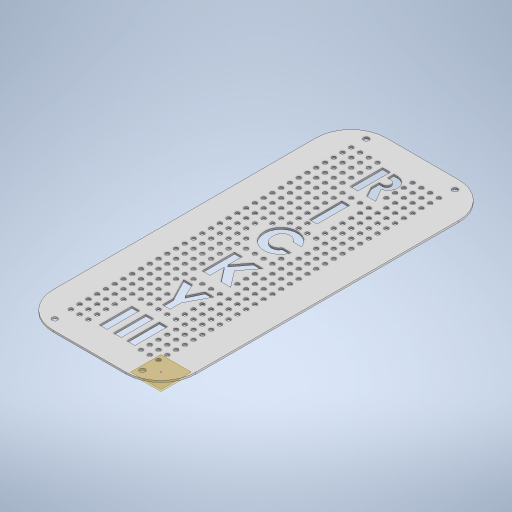
# Autodesk Inventor part: Ground Station cover
Saved by Autodesk Inventor 2023 (Build 270158000, 158)
## iProperties
Created: 2023-02-28
Part Number: Ground Station cover
Material: Generic
Document SubType Name: Modeling
Designer: mikep
Density: 1 g/cm^3
Appearance: Default
Author: mikep
Autodesk Inventor part; units mm, degrees
ref_plane "YZ Plane" through (0, 0, 0) normal (1, 0, 0) x (0, 1, 0)
ref_plane "XZ Plane" through (0, 0, 0) normal (0, 1, 0) x (-1, 0, 0)
ref_plane "XY Plane" through (0, 0, 0) normal (0, 0, 1) x (1, 0, 0)
ref_plane "Work Plane1" through (0, 12.7, 0) normal (0, 1, 0) x (1, 0, 0)
sketch "Sketch5" plane through (0, 12.7, 0) normal (0, 1, 0) x (1, 0, 0)
  line L0 (-90.805, -12.7) -> (12.7, -12.7)
  line L1 (12.7, -12.7) -> (12.7, 228.6)
  line L2 (12.7, 228.6) -> (-90.805, 228.6)
  line L3 (-90.805, 228.6) -> (-90.805, -12.7)
  line L4 (0, 0) -> (0, 215.9) projected
  line L5 (0, 215.9) -> (-78.105, 215.9) projected
  dimension "d18" = 241.3
  dimension "d19" = 103.505
  dimension "d20" = 12.7
  dimension "d21" = 12.7
  constraints: 8 end point, 2 parallel, 1 horizontal, 1 perpendicular
  measures "d18" distance of L1.end L0.end
  measures "d19" distance of L1.end L2.end
  measures "d20" distance between parallel lines of L1 L4
  measures "d21" distance between parallel lines of L5 L2
extrude "Extrusion4" add sketch "Sketch5" along normal blind 1.27
sketch "Sketch6" plane through (0, 13.97, 0) normal (0, 1, 0) x (1, 0, 0)
  point P0 (0, 0)
ref_plane "Work Plane3" through (0, 13.97, 0) normal (0, 1, 0) x (1, 0, 0)
sketch "Sketch8" plane through (0, 13.97, 0) normal (0, 1, 0) x (1, 0, 0)
  line L0 (-74.295, 3.81) -> (-3.81, 3.81) projected
  line L1 (-51.8748, 30.8065) -> (-46.268, 30.8065)
  line L2 (-46.268, 30.8065) -> (-46.268, 7.3025)
  line L3 (-46.268, 7.3025) -> (-51.8748, 7.3025)
  line L4 (-51.8748, 7.3025) -> (-51.8748, 30.8065)
  line L5 (-41.6807, 30.8065) -> (-36.074, 30.8065)
  line L6 (-36.074, 30.8065) -> (-36.074, 7.3025)
  line L7 (-36.074, 7.3025) -> (-41.6807, 7.3025)
  line L8 (-41.6807, 7.3025) -> (-41.6807, 30.8065)
  line L9 (-31.9235, 30.8065) -> (-26.0983, 30.8065)
  line L10 (-26.0983, 30.8065) -> (-26.0983, 7.3025)
  line L11 (-26.0983, 7.3025) -> (-31.9235, 7.3025)
  line L12 (-31.9235, 7.3025) -> (-31.9235, 30.8065)
  line L13 (-41.6192, 42.7474) -> (-36.1235, 42.7474)
  line L14 (-36.1235, 42.7474) -> (-36.1235, 50.6586)
  line L15 (-36.1235, 50.6586) -> (-27.9507, 66.2951)
  line L16 (-27.9507, 66.2951) -> (-34.288, 66.2951)
  line L17 (-34.288, 66.2951) -> (-38.8713, 56.5194)
  line L18 (-38.8713, 56.5194) -> (-43.4546, 66.2951)
  line L19 (-43.4546, 66.2951) -> (-49.7919, 66.2951)
  line L20 (-49.7919, 66.2951) -> (-41.6192, 50.6586)
  line L21 (-41.6192, 50.6586) -> (-41.6192, 42.7474)
  line L22 (-48.5981, 101.9465) -> (-48.5981, 78.5001)
  line L23 (-48.5981, 78.5001) -> (-42.9914, 78.5001)
  line L24 (-42.9914, 78.5001) -> (-42.9914, 88.9127)
  line L25 (-42.9914, 88.9127) -> (-34.9817, 78.5001)
  line L26 (-34.9817, 78.5001) -> (-27.9507, 78.5001)
  line L27 (-27.9507, 78.5001) -> (-36.9685, 90.2233)
  line L28 (-36.9685, 90.2233) -> (-27.9507, 101.9465)
  line L29 (-27.9507, 101.9465) -> (-34.9817, 101.9465)
  line L30 (-34.9817, 101.9465) -> (-42.9914, 91.534)
  line L31 (-42.9914, 91.534) -> (-42.9914, 101.9465)
  line L32 (-42.9914, 101.9465) -> (-48.5981, 101.9465)
  line L33 (-27.6673, 121.9946) -> (-33.9997, 121.9946)
  arc A0 (-44.2292, 129.1064) -> (-44.1364, 122.3681) centre (-36.4286, 125.844) ccw
  line L34 (-33.8768, 129.6183) -> (-27.6561, 129.6183)
  arc A1 (-44.1364, 122.3681) -> (-33.9997, 121.9946) centre (-38.9754, 124.6955) ccw
  arc A2 (-33.8768, 129.6183) -> (-44.2292, 129.1064) centre (-38.9307, 126.8905) ccw
  arc A3 (-27.6561, 129.6183) -> (-50.2579, 129.6183) centre (-38.957, 125.9562) ccw
  arc A4 (-50.2579, 129.6183) -> (-50.2881, 122.3885) centre (-38.957, 125.9562) ccw
  arc A5 (-50.2881, 122.3885) -> (-27.6673, 121.9946) centre (-38.9225, 125.3595) ccw
  line L35 (-41.8513, 173.0184) -> (-36.3002, 173.0184)
  line L36 (-36.3002, 173.0184) -> (-36.3002, 149.5617)
  line L37 (-36.3002, 149.5617) -> (-41.8513, 149.5617)
  line L38 (-41.8513, 149.5617) -> (-41.8513, 173.0184)
  line L39 (-47.9527, 208.5865) -> (-47.9527, 185.035)
  line L40 (-47.9527, 185.035) -> (-42.2829, 185.035)
  line L41 (-42.2829, 185.035) -> (-42.2829, 194.0541)
  line L42 (-39.7429, 192.064) -> (-35.8412, 185.035)
  line L43 (-35.8412, 185.035) -> (-29.3552, 185.035)
  line L44 (-29.3552, 185.035) -> (-34.8878, 194.4069)
  arc A6 (-34.8878, 194.4069) -> (-34.8878, 208.176) centre (-36.7536, 201.2914) ccw
  arc A7 (-34.8878, 208.176) -> (-37.3133, 208.5865) centre (-38.2098, 195.9186) ccw
  line L45 (-42.2829, 203.9834) -> (-42.2829, 197.929)
  line L46 (-39.7429, 197.929) -> (-37.2678, 197.929)
  line L47 (-39.7429, 203.9834) -> (-37.2678, 203.9834)
  arc A8 (-37.2678, 197.929) -> (-37.2678, 203.9834) centre (-37.2678, 200.9562) ccw
  line L48 (-42.2829, 194.0541) -> (-42.2829, 197.929)
  line L49 (-39.7429, 192.064) -> (-39.7429, 197.929)
  line L50 (-42.2829, 203.9834) -> (-42.2829, 208.5865)
  line L51 (-39.7429, 208.5865) -> (-39.7429, 203.9834)
  line L52 (-47.9527, 208.5865) -> (-42.2829, 208.5865)
  line L53 (-39.7429, 208.5865) -> (-37.3133, 208.5865)
  line L54 (-90.805, 228.6) -> (-90.805, -12.7) projected
  line L55 (-90.805, 107.95) -> (12.7, 107.95) construction
  line L56 (12.7, -12.7) -> (12.7, 228.6) projected
  line L57 (12.7, 228.6) -> (-90.805, 228.6) projected
  line L58 (-39.0525, 228.6) -> (-39.0525, -12.7) construction
  line L59 (-90.805, -12.7) -> (12.7, -12.7) projected
  point P0 (0, 0)
  point P1 (-31.9235, 3.81)
  point P2 (-51.8748, 3.81)
  point P3 (-41.6807, 3.81)
  point P4 (-26.0983, 3.81)
  point P5 (-46.268, 3.81)
  point P6 (-36.074, 3.81)
  dimension "d54" = 2.54
  dimension "d55" = 2.54
  constraints: 110 end point, 19 point on circle, 14 perpendicular, 13 parallel, 11 horizontal, 11 point on line, 9 centre point, 5 tangent, 4 equal length, 4 midpoint, 4 vertical, 1 concentric
  measures "d54" distance from line of L49 L45.end
  measures "d55" distance between parallel lines of L50 L51
extrude "Extrusion5" cut sketch "Sketch8" against normal blind 25.4 contours L1 L2 L3 L4 | L5 L6 L7 L8 | L9 L10 L11 L12 | L21 L20 L19 L18 L17 L16 L15 L14 L13 | L32 L31 L30 L29 L28 L27 L26 L25 L24 L23 L22 | A5 A4 A3 L34 A2 A0 A1 L33 | L35 L36 L37 L38 | L52 L50 L45 L48 L41 L40 L39 | L49 L46 A8 L47 L51 L53 A7 A6 L44 L43 L42
ref_plane "Work Plane2" through (0, 13.97, 0) normal (0, 1, 0) x (1, 0, 0)
sketch "Sketch9" plane through (0, 13.97, 0) normal (0, 1, 0) x (1, 0, 0)
  line L0 (-3.81, 212.09) -> (-74.295, 212.09) construction
  line L1 (-74.295, 212.09) -> (-3.81, 212.09) construction
  line L2 (-3.81, 212.09) -> (-74.295, 212.09) construction
  line L3 (-74.295, 212.09) -> (-74.295, 22.9425) construction
  line L4 (-74.295, 3.81) -> (-3.81, 3.81) construction
  line L5 (-71.9663, 3.81) -> (-6.4229, 3.81) construction
  point P0 (0, 0)
  point P1 (-71.9663, 209.9147)
  point P2 (-71.9663, 203.5647)
  point P3 (-71.9663, 197.2147)
  point P4 (-71.9663, 190.8647)
  point P5 (-71.9663, 184.5147)
  point P6 (-71.9663, 178.1647)
  point P7 (-71.9663, 171.8147)
  point P8 (-71.9663, 165.4647)
  point P9 (-71.9663, 159.1147)
  point P10 (-71.9663, 152.7647)
  point P11 (-71.9663, 146.4147)
  point P12 (-71.9663, 140.0647)
  point P13 (-71.9663, 133.7147)
  point P14 (-71.9663, 127.3647)
  point P15 (-71.9663, 121.0147)
  point P16 (-71.9663, 114.6647)
  point P17 (-71.9663, 108.3147)
  point P18 (-71.9663, 101.9647)
  point P19 (-71.9663, 95.6147)
  point P20 (-71.9663, 89.2647)
  point P21 (-71.9663, 82.9147)
  point P22 (-71.9663, 76.5647)
  point P23 (-71.9663, 70.2147)
  point P24 (-71.9663, 63.8647)
  point P25 (-71.9663, 57.5147)
  point P26 (-71.9663, 51.1647)
  point P27 (-71.9663, 44.8147)
  point P28 (-71.9663, 38.4647)
  point P29 (-71.9663, 32.1147)
  point P30 (-71.9663, 25.7647)
  point P31 (-71.9663, 19.4147)
  point P32 (-71.9663, 13.0647)
  point P33 (-71.9663, 6.7147)
  point P34 (-65.6163, 209.9147)
  point P35 (-65.6163, 203.5647)
  point P36 (-65.6163, 197.2147)
  point P37 (-65.6163, 190.8647)
  point P38 (-65.6163, 184.5147)
  point P39 (-65.6163, 178.1647)
  point P40 (-65.6163, 171.8147)
  point P41 (-65.6163, 165.4647)
  point P42 (-65.6163, 159.1147)
  point P43 (-65.6163, 152.7647)
  point P44 (-65.6163, 146.4147)
  point P45 (-65.6163, 140.0647)
  point P46 (-65.6163, 133.7147)
  point P47 (-65.6163, 127.3647)
  point P48 (-65.6163, 121.0147)
  point P49 (-65.6163, 114.6647)
  point P50 (-65.6163, 108.3147)
  point P51 (-65.6163, 101.9647)
  point P52 (-65.6163, 95.6147)
  point P53 (-65.6163, 89.2647)
  point P54 (-65.6163, 82.9147)
  point P55 (-65.6163, 76.5647)
  point P56 (-65.6163, 70.2147)
  point P57 (-65.6163, 63.8647)
  point P58 (-65.6163, 57.5147)
  point P59 (-65.6163, 51.1647)
  point P60 (-65.6163, 44.8147)
  point P61 (-65.6163, 38.4647)
  point P62 (-65.6163, 32.1147)
  point P63 (-65.6163, 25.7647)
  point P64 (-65.6163, 19.4147)
  point P65 (-65.6163, 13.0647)
  point P66 (-65.6163, 6.7147)
  point P67 (-59.2663, 209.9147)
  point P68 (-59.2663, 203.5647)
  point P69 (-59.2663, 197.2147)
  point P70 (-59.2663, 190.8647)
  point P71 (-59.2663, 184.5147)
  point P72 (-59.2663, 178.1647)
  point P73 (-59.2663, 171.8147)
  point P74 (-59.2663, 165.4647)
  point P75 (-59.2663, 159.1147)
  point P76 (-59.2663, 152.7647)
  point P77 (-59.2663, 146.4147)
  point P78 (-59.2663, 140.0647)
  point P79 (-59.2663, 133.7147)
  point P80 (-59.2663, 127.3647)
  point P81 (-59.2663, 121.0147)
  point P82 (-59.2663, 114.6647)
  point P83 (-59.2663, 108.3147)
  point P84 (-59.2663, 101.9647)
  point P85 (-59.2663, 95.6147)
  point P86 (-59.2663, 89.2647)
  point P87 (-59.2663, 82.9147)
  point P88 (-59.2663, 76.5647)
  point P89 (-59.2663, 70.2147)
  point P90 (-59.2663, 63.8647)
  point P91 (-59.2663, 57.5147)
  point P92 (-59.2663, 51.1647)
  point P93 (-59.2663, 44.8147)
  point P94 (-59.2663, 38.4647)
  point P95 (-59.2663, 32.1147)
  point P96 (-59.2663, 25.7647)
  point P97 (-59.2663, 19.4147)
  point P98 (-59.2663, 13.0647)
  point P99 (-59.2663, 6.7147)
  point P100 (-52.9163, 209.9147)
  point P101 (-52.9163, 203.5647)
  point P102 (-52.9163, 197.2147)
  point P103 (-52.9163, 190.8647)
  point P104 (-52.9163, 184.5147)
  point P105 (-52.9163, 178.1647)
  point P106 (-52.9163, 171.8147)
  point P107 (-52.9163, 165.4647)
  point P108 (-52.9163, 159.1147)
  point P109 (-52.9163, 152.7647)
  point P110 (-52.9163, 146.4147)
  point P111 (-52.9163, 140.0647)
  point P112 (-52.9163, 133.7147)
  point P113 (-52.9163, 114.6647)
  point P114 (-52.9163, 108.3147)
  point P115 (-52.9163, 101.9647)
  point P116 (-52.9163, 95.6147)
  point P117 (-52.9163, 89.2647)
  point P118 (-52.9163, 82.9147)
  point P119 (-52.9163, 76.5647)
  point P120 (-52.9163, 70.2147)
  point P121 (-52.9163, 63.8647)
  point P122 (-52.9163, 57.5147)
  point P123 (-52.9163, 51.1647)
  point P124 (-52.9163, 44.8147)
  point P125 (-52.9163, 38.4647)
  point P126 (-52.9163, 25.7647)
  point P127 (-52.9163, 19.4147)
  point P128 (-52.9163, 13.0647)
  point P129 (-52.9163, 6.7147)
  point P130 (-46.5663, 203.5647)
  point P131 (-46.5663, 197.2147)
  point P132 (-46.5663, 190.8647)
  point P133 (-46.5663, 184.5147)
  point P134 (-46.5663, 178.1647)
  point P135 (-46.5663, 171.8147)
  point P136 (-46.5663, 165.4647)
  point P137 (-46.5663, 159.1147)
  point P138 (-46.5663, 152.7647)
  point P139 (-46.5663, 146.4147)
  point P140 (-46.5663, 140.0647)
  point P141 (-46.5663, 133.7147)
  point P142 (-46.5663, 127.3647)
  point P143 (-46.5663, 121.0147)
  point P144 (-46.5663, 114.6647)
  point P145 (-46.5663, 108.3147)
  point P146 (-46.5663, 101.9647)
  point P147 (-46.5663, 95.6147)
  point P148 (-46.5663, 89.2647)
  point P149 (-46.5663, 82.9147)
  point P150 (-46.5663, 70.2147)
  point P151 (-46.5663, 63.8647)
  point P152 (-46.5663, 51.1647)
  point P153 (-46.5663, 44.8147)
  point P154 (-46.5663, 38.4647)
  point P155 (-46.5663, 25.7647)
  point P156 (-46.5663, 19.4147)
  point P157 (-46.5663, 13.0647)
  point P158 (-46.5663, 6.7147)
  point P159 (-40.2163, 203.5647)
  point P160 (-40.2163, 197.2147)
  point P161 (-40.2163, 190.8647)
  point P162 (-40.2163, 178.1647)
  point P163 (-40.2163, 171.8147)
  point P164 (-40.2163, 165.4647)
  point P165 (-40.2163, 159.1147)
  point P166 (-40.2163, 152.7647)
  point P167 (-40.2163, 146.4147)
  point P168 (-40.2163, 140.0647)
  point P169 (-40.2163, 133.7147)
  point P170 (-40.2163, 114.6647)
  point P171 (-40.2163, 108.3147)
  point P172 (-40.2163, 101.9647)
  point P173 (-40.2163, 95.6147)
  point P174 (-40.2163, 89.2647)
  point P175 (-40.2163, 82.9147)
  point P176 (-40.2163, 70.2147)
  point P177 (-40.2163, 63.8647)
  point P178 (-40.2163, 57.5147)
  point P179 (-40.2163, 51.1647)
  point P180 (-40.2163, 44.8147)
  point P181 (-40.2163, 38.4647)
  point P182 (-40.2163, 25.7647)
  point P183 (-40.2163, 19.4147)
  point P184 (-40.2163, 13.0647)
  point P185 (-40.2163, 6.7147)
  point P186 (-33.8663, 203.5647)
  point P187 (-33.8663, 197.2147)
  point P188 (-33.8663, 190.8647)
  point P189 (-33.8663, 184.5147)
  point P190 (-33.8663, 178.1647)
  point P191 (-33.8663, 140.0647)
  point P192 (-33.8663, 133.7147)
  point P193 (-33.8663, 121.0147)
  point P194 (-33.8663, 114.6647)
  point P195 (-33.8663, 108.3147)
  point P196 (-33.8663, 101.9647)
  point P197 (-33.8663, 95.6147)
  point P198 (-33.8663, 89.2647)
  point P199 (-33.8663, 82.9147)
  dimension "d48" = 6.35
  dimension "d51" = 6.35
  constraints: 8 end point, 2 horizontal, 2 point on line, 1 collinear, 1 vertical, 313 other
  measures "d48" distance of point (-71.966, 209.915) point (-71.966, 203.565)
  measures "d51" distance of point (-71.966, 209.915) point (-65.616, 209.915)
hole "Hole1" at (-65.6163, 13.97, -209.9147) at (-71.9663, 13.97, -209.9147) at (-59.2663, 13.97, -209.9147) at (-52.9163, 13.97, -209.9147) at (-27.5163, 13.97, -209.9147) at (-21.1663, 13.97, -209.9147) at (-14.8163, 13.97, -209.9147) at (-8.4663, 13.97, -209.9147) at (-8.4663, 13.97, -203.5647) at (-14.8163, 13.97, -203.5647) at (-21.1663, 13.97, -203.5647) at (-27.5163, 13.97, -203.5647) at (-52.9163, 13.97, -203.5647) at (-59.2663, 13.97, -203.5647) at (-65.6163, 13.97, -203.5647) at (-71.9663, 13.97, -203.5647) at (-71.9663, 13.97, -197.2147) at (-65.6163, 13.97, -197.2147) at (-59.2663, 13.97, -197.2147) at (-52.9163, 13.97, -197.2147) at (-27.5163, 13.97, -197.2147) at (-21.1663, 13.97, -197.2147) at (-14.8163, 13.97, -197.2147) at (-8.4663, 13.97, -197.2147) at (-8.4663, 13.97, -190.8647) at (-14.8163, 13.97, -190.8647) at (-21.1663, 13.97, -190.8647) at (-27.5163, 13.97, -190.8647) at (-52.9163, 13.97, -190.8647) at (-59.2663, 13.97, -190.8647) at (-65.6163, 13.97, -190.8647) at (-71.9663, 13.97, -190.8647) at (-71.9663, 13.97, -184.5147) at (-65.6163, 13.97, -184.5147) at (-59.2663, 13.97, -184.5147) at (-52.9163, 13.97, -184.5147) at (-21.1663, 13.97, -184.5147) at (-14.8163, 13.97, -184.5147) at (-8.4663, 13.97, -184.5147) at (-8.4663, 13.97, -178.1647) at (-14.8163, 13.97, -178.1647) at (-21.1663, 13.97, -178.1647) at (-27.5163, 13.97, -178.1647) at (-33.8663, 13.97, -178.1647) at (-40.2163, 13.97, -178.1647) at (-46.5663, 13.97, -178.1647) at (-52.9163, 13.97, -178.1647) at (-59.2663, 13.97, -178.1647) at (-65.6163, 13.97, -178.1647) at (-71.9663, 13.97, -178.1647) direction (0, -1, 0) diameter 3 depth 19.05 tip angle 118 and at (-71.9663, 13.97, -171.8147) (-65.6163, 13.97, -171.8147) (-59.2663, 13.97, -171.8147) (-52.9163, 13.97, -171.8147) (-46.5663, 13.97, -171.8147) (-27.5163, 13.97, -171.8147) (-21.1663, 13.97, -171.8147) (-14.8163, 13.97, -171.8147) (-8.4663, 13.97, -171.8147) (-8.4663, 13.97, -165.4647) (-14.8163, 13.97, -165.4647) (-21.1663, 13.97, -165.4647) (-27.5163, 13.97, -165.4647) (-46.5663, 13.97, -165.4647) (-52.9163, 13.97, -165.4647) (-59.2663, 13.97, -165.4647) (-65.6163, 13.97, -165.4647) (-71.9663, 13.97, -165.4647) (-71.9663, 13.97, -159.1147) (-65.6163, 13.97, -159.1147) (-59.2663, 13.97, -159.1147) (-52.9163, 13.97, -159.1147) (-46.5663, 13.97, -159.1147) (-27.5163, 13.97, -159.1147) (-21.1663, 13.97, -159.1147) (-14.8163, 13.97, -159.1147) (-8.4663, 13.97, -159.1147) (-8.4663, 13.97, -152.7647) (-14.8163, 13.97, -152.7647) (-21.1663, 13.97, -152.7647) (-27.5163, 13.97, -152.7647) (-46.5663, 13.97, -152.7647) (-52.9163, 13.97, -152.7647) (-59.2663, 13.97, -152.7647) (-65.6163, 13.97, -152.7647) (-71.9663, 13.97, -152.7647) (-71.9663, 13.97, -146.4147) (-65.6163, 13.97, -146.4147) (-59.2663, 13.97, -146.4147) (-52.9163, 13.97, -146.4147) (-46.5663, 13.97, -146.4147) (-40.2163, 13.97, -146.4147) (-27.5163, 13.97, -146.4147) (-21.1663, 13.97, -146.4147) (-14.8163, 13.97, -146.4147) (-8.4663, 13.97, -146.4147) (-8.4663, 13.97, -140.0647) (-14.8163, 13.97, -140.0647) (-21.1663, 13.97, -140.0647) (-27.5163, 13.97, -140.0647) (-33.8663, 13.97, -140.0647) (-40.2163, 13.97, -140.0647) (-46.5663, 13.97, -140.0647) (-52.9163, 13.97, -140.0647) (-59.2663, 13.97, -140.0647) (-65.6163, 13.97, -140.0647) (-71.9663, 13.97, -140.0647) (-71.9663, 13.97, -133.7147) (-65.6163, 13.97, -133.7147) (-59.2663, 13.97, -133.7147) (-52.9163, 13.97, -133.7147) (-21.1663, 13.97, -133.7147) (-14.8163, 13.97, -133.7147) (-8.4663, 13.97, -133.7147) (-8.4663, 13.97, -127.3647) (-14.8163, 13.97, -127.3647) (-21.1663, 13.97, -127.3647) (-59.2663, 13.97, -127.3647) (-65.6163, 13.97, -127.3647) (-71.9663, 13.97, -127.3647) (-71.9663, 13.97, -121.0147) (-65.6163, 13.97, -121.0147) (-59.2663, 13.97, -121.0147) (-21.1663, 13.97, -121.0147) (-14.8163, 13.97, -121.0147) (-8.4663, 13.97, -121.0147) (-8.4663, 13.97, -114.6647) (-14.8163, 13.97, -114.6647) (-21.1663, 13.97, -114.6647) (-27.5163, 13.97, -114.6647) (-52.9163, 13.97, -114.6647) (-59.2663, 13.97, -114.6647) (-65.6163, 13.97, -114.6647) (-71.9663, 13.97, -114.6647) (-71.9663, 13.97, -108.3147) (-65.6163, 13.97, -108.3147) (-59.2663, 13.97, -108.3147) (-52.9163, 13.97, -108.3147) (-46.5663, 13.97, -108.3147) (-40.2163, 13.97, -108.3147) (-33.8663, 13.97, -108.3147) (-27.5163, 13.97, -108.3147) (-21.1663, 13.97, -108.3147) (-14.8163, 13.97, -108.3147) (-8.4663, 13.97, -108.3147) (-8.4663, 13.97, -101.9647) (-14.8163, 13.97, -101.9647) (-21.1663, 13.97, -101.9647) (-52.9163, 13.97, -101.9647) (-59.2663, 13.97, -101.9647) (-65.6163, 13.97, -101.9647) (-71.9663, 13.97, -101.9647) (-71.9663, 13.97, -95.6147) (-65.6163, 13.97, -95.6147) (-59.2663, 13.97, -95.6147) (-52.9163, 13.97, -95.6147) (-27.5163, 13.97, -95.6147) (-21.1663, 13.97, -95.6147) (-14.8163, 13.97, -95.6147) (-8.4663, 13.97, -95.6147) (-8.4663, 13.97, -89.2647) (-14.8163, 13.97, -89.2647) (-21.1663, 13.97, -89.2647) (-27.5163, 13.97, -89.2647) (-52.9163, 13.97, -89.2647) (-59.2663, 13.97, -89.2647) (-65.6163, 13.97, -89.2647) (-71.9663, 13.97, -89.2647) (-71.9663, 13.97, -82.9147) (-65.6163, 13.97, -82.9147) (-59.2663, 13.97, -82.9147) (-52.9163, 13.97, -82.9147) (-27.5163, 13.97, -82.9147) (-21.1663, 13.97, -82.9147) (-14.8163, 13.97, -82.9147) (-8.4663, 13.97, -82.9147) (-14.8163, 13.97, -76.5647) (-8.4663, 13.97, -76.5647) (-21.1663, 13.97, -76.5647) (-52.9163, 13.97, -76.5647) (-59.2663, 13.97, -76.5647) (-65.6163, 13.97, -76.5647) (-71.9663, 13.97, -76.5647) (-71.9663, 13.97, -70.2147) (-65.6163, 13.97, -70.2147) (-59.2663, 13.97, -70.2147) (-52.9163, 13.97, -70.2147) (-46.5663, 13.97, -70.2147) (-40.2163, 13.97, -70.2147) (-33.8663, 13.97, -70.2147) (-27.5163, 13.97, -70.2147) (-21.1663, 13.97, -70.2147) (-14.8163, 13.97, -70.2147) (-8.4663, 13.97, -70.2147) (-8.4663, 13.97, -63.8647) (-14.8163, 13.97, -63.8647) (-21.1663, 13.97, -63.8647) (-52.9163, 13.97, -63.8647) (-59.2663, 13.97, -63.8647) (-65.6163, 13.97, -63.8647) (-71.9663, 13.97, -63.8647) (-71.9663, 13.97, -57.5147) (-65.6163, 13.97, -57.5147) (-59.2663, 13.97, -57.5147) (-52.9163, 13.97, -57.5147) (-27.5163, 13.97, -57.5147) (-21.1663, 13.97, -57.5147) (-14.8163, 13.97, -57.5147) (-8.4663, 13.97, -57.5147) (-8.4663, 13.97, -51.1647) (-14.8163, 13.97, -51.1647) (-21.1663, 13.97, -51.1647) (-27.5163, 13.97, -51.1647) (-46.5663, 13.97, -51.1647) (-52.9163, 13.97, -51.1647) (-59.2663, 13.97, -51.1647) (-65.6163, 13.97, -51.1647) (-71.9663, 13.97, -51.1647) (-71.9663, 13.97, -44.8147) (-65.6163, 13.97, -44.8147) (-59.2663, 13.97, -44.8147) (-52.9163, 13.97, -44.8147) (-46.5663, 13.97, -44.8147) (-27.5163, 13.97, -44.8147) (-21.1663, 13.97, -44.8147) (-14.8163, 13.97, -44.8147) (-8.4663, 13.97, -44.8147) (-8.4663, 13.97, -38.4647) (-14.8163, 13.97, -38.4647) (-21.1663, 13.97, -38.4647) (-27.5163, 13.97, -38.4647) (-33.8663, 13.97, -38.4647) (-40.2163, 13.97, -38.4647) (-46.5663, 13.97, -38.4647) (-52.9163, 13.97, -38.4647) (-59.2663, 13.97, -38.4647) (-65.6163, 13.97, -38.4647) (-71.9663, 13.97, -38.4647) (-71.9663, 13.97, -32.1147) (-65.6163, 13.97, -32.1147) (-59.2663, 13.97, -32.1147) (-21.1663, 13.97, -32.1147) (-14.8163, 13.97, -32.1147) (-8.4663, 13.97, -32.1147) (-8.4663, 13.97, -25.7647) (-14.8163, 13.97, -25.7647) (-21.1663, 13.97, -25.7647) (-59.2663, 13.97, -25.7647) (-65.6163, 13.97, -25.7647) (-71.9663, 13.97, -25.7647) (-71.9663, 13.97, -19.4147) (-65.6163, 13.97, -19.4147) (-59.2663, 13.97, -19.4147) (-71.9663, 13.97, -13.0647) (-65.6163, 13.97, -13.0647) (-59.2663, 13.97, -13.0647) (-71.9663, 13.97, -6.7147) (-65.6163, 13.97, -6.7147) (-59.2663, 13.97, -6.7147) (-21.1663, 13.97, -13.0647) (-21.1663, 13.97, -19.4147) (-14.8163, 13.97, -19.4147) (-8.4663, 13.97, -19.4147) (-8.4663, 13.97, -13.0647) (-14.8163, 13.97, -13.0647) (-21.1663, 13.97, -6.7147) (-8.4663, 13.97, -6.7147) (-14.8163, 13.97, -6.7147)
sketch "Sketch10" plane through (0, 13.97, 0) normal (0, 1, 0) x (1, 0, 0)
  line L0 (12.7, 228.6) -> (-90.805, 228.6) projected
  line L1 (-90.805, -12.7) -> (12.7, -12.7) projected
  point P0 (0, 0)
  point P1 (-7.9517, 220.98)
  point P2 (-71.8565, -5.08)
  point P3 (-71.8565, 220.6612)
  point P4 (-7.8772, -5.5099)
  dimension "d56" = 7.62
  dimension "d57" = 7.62
  measures "d56" distance from line of point (-71.857, -5.08) L1
  measures "d57" distance from line of point (-7.952, 220.98) L0
hole "Hole2" at (-7.9517, 13.97, -220.98) at (-71.8565, 13.97, 5.08) at (-71.8565, 13.97, -220.6612) at (-7.8772, 13.97, 5.5099) direction (0, -1, 0) diameter 4 depth 19.05 tip angle 118
fillet "Fillet1" radius 25.4 4 edges at (-90.805, 13.335, -228.6) (12.7, 13.335, -228.6) (12.7, 13.335, 12.7) (-90.805, 13.335, 12.7)
body "Solid1"
